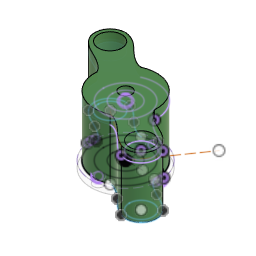
LED_clamp_fiber_mount_C20A10H740 v2 (Autodesk Fusion 360 design; units mm, degrees)
Autodesk Fusion 360 part; units mm, degrees
sketch "Sketch1" plane through (0, 0, 0) normal (0, 0, 1) x (1, 0, 0) in component "C20A1-H740-30"
  circle A0 centre (0, 0) radius 10
  line L0 (-10, 0) -> (10, 0) construction
  arc A1 (-9.9306, -1.1764) -> (-9.9306, 1.1764) centre (-10, 0) ccw
  line L1 (0, 0) -> (0, 5.1489) construction
  arc A2 (9.9306, 1.1764) -> (9.9306, -1.1764) centre (10, 0) ccw
  circle A3 centre (0, 7.8996) radius 1.5
  circle A4 centre (0, -7.8996) radius 1.5
  dimension "d4" = 20
  dimension "d8" = 3
  constraint coincident A0.centre L1.start
  constraint coincident A0 L0.start
  constraint coincident A0 L0.end
  constraint horizontal L0
  constraint coincident A0.centre L0
  constraint coincident A0 A1.start
  constraint coincident A0 A1.end
  constraint coincident L0.start A1.centre
  constraint perpendicular L0 L1
  constraint symmetric A1.start L1 A2.end
  constraint symmetric A1.end L1 A2.start
  constraint symmetric A1 L1 A2
  constraint coincident L1 A3.centre
  constraint symmetric L0 A3 A4
  measures "d4" diameter of A0
  measures "d8" diameter of A3
extrude "Extrude1" add sketch "Sketch1" along normal blind 1.9 contours A0 A1 A2 makes body 1 in component "C20A1-H740-30"
sketch "Sketch1 (2)" plane through (0, 0, 1.9) normal (0, 0, 1) x (-1, 0, 0) in component "optic fiber mount"
  circle A0 centre (0, -7.8996) radius 1.5 construction
  circle A1 centre (0, 7.8996) radius 1.5 construction
  arc A2 (9.9306, 1.1764) -> (-9.9306, 1.1764) centre (0, 0) ccw construction
  arc A3 (-9.9306, -1.1764) -> (-9.9306, 1.1764) centre (-10, 0) ccw construction
  arc A4 (-9.9306, -1.1764) -> (9.9306, -1.1764) centre (0, 0) ccw construction
  arc A5 (9.9306, 1.1764) -> (9.9306, -1.1764) centre (10, 0) ccw construction
  line L0 (12.7, -9.5942) -> (-12.7, -9.5942) construction
  line L1 (0, 0) -> (0, -1.0835) construction
  line L2 (0, -1.0835) -> (0, -4.3356) construction
  line L3 (0, 0) -> (-4.8971, 0) construction
  circle A6 centre (12.7, -9.5942) radius 3.429
  circle A7 centre (-12.7, -9.5942) radius 3.429
  circle A8 centre (0, 0) radius 1.8
  circle A9 centre (0, 0) radius 9
  circle A10 centre (0, 0) radius 6.46
  circle A11 centre (0, 0) radius 3.8
  spline S0 degree 5 poles (14.5589, -5.5565) (14.3535, -5.462) (13.9487, -5.267) (13.3592, -4.9569) (12.6123, -4.5075) (11.7634, -3.8821) (11.0225, -3.1882) (10.4081, -2.4217) (9.9244, -1.5822) (9.5489, -0.6771) (9.2444, 0.2825) (9.0258, 1.0848) (8.8613, 1.702) (8.7495, 2.12) (8.693, 2.3306) knots 0 0 0 0 0 0 0.1 0.2 0.3 0.4 0.5 0.6 0.7 0.8 0.9 1 1 1 1 1 1
  line L4 (0, 0) -> (12.7, -9.5942) construction
  spline S1 degree 5 poles (9.3242, -12.4858) (9.1771, -12.3141) (8.8789, -11.978) (8.4194, -11.4957) (7.783, -10.9001) (6.9494, -10.2544) (6.0795, -9.7314) (5.1742, -9.3499) (4.2345, -9.1141) (3.2612, -9.0002) (2.2549, -8.9696) (1.4234, -8.9786) (0.7847, -8.9891) (0.3521, -8.9958) (0.1341, -8.999) knots 0 0 0 0 0 0 0.1 0.2 0.3 0.4 0.5 0.6 0.7 0.8 0.9 1 1 1 1 1 1
  line L5 (15.6873, -6.0761) -> (13.4304, -5.037)
  line L6 (9.0147, 1.1306) -> (8.3713, 3.5305)
  line L7 (10.1323, -13.4293) -> (8.516, -11.5423)
  line L8 (1.3763, -8.9805) -> (-1.1081, -9.0175)
  arc A12 (9.3242, -12.4858) -> (14.5589, -5.5565) centre (12.7, -9.5942) ccw
  spline S2 degree 5 poles (-14.5589, -5.5565) (-14.3535, -5.462) (-13.9487, -5.267) (-13.3592, -4.9569) (-12.6123, -4.5075) (-11.7634, -3.8821) (-11.0225, -3.1882) (-10.4081, -2.4217) (-9.9244, -1.5822) (-9.5489, -0.6771) (-9.2444, 0.2825) (-9.0258, 1.0848) (-8.8613, 1.702) (-8.7495, 2.12) (-8.693, 2.3306) knots 0 0 0 0 0 0 0.1 0.2 0.3 0.4 0.5 0.6 0.7 0.8 0.9 1 1 1 1 1 1
  line L9 (-15.6873, -6.0761) -> (-13.4304, -5.037)
  line L10 (-9.0147, 1.1306) -> (-8.3713, 3.5305)
  spline S3 degree 5 poles (-9.3242, -12.4858) (-9.1771, -12.3141) (-8.8789, -11.978) (-8.4194, -11.4957) (-7.783, -10.9001) (-6.9494, -10.2544) (-6.0795, -9.7314) (-5.1742, -9.3499) (-4.2345, -9.1141) (-3.2612, -9.0002) (-2.2549, -8.9696) (-1.4234, -8.9786) (-0.7847, -8.9891) (-0.3521, -8.9958) (-0.1341, -8.999) knots 0 0 0 0 0 0 0.1 0.2 0.3 0.4 0.5 0.6 0.7 0.8 0.9 1 1 1 1 1 1
  line L11 (-10.1323, -13.4293) -> (-8.516, -11.5423)
  line L12 (-1.3763, -8.9805) -> (1.1081, -9.0175)
  arc A13 (-14.5589, -5.5565) -> (-9.3242, -12.4858) centre (-12.7, -9.5942) ccw
  point P0 (0, -9.5942)
  point P1 (10.4158, -2.3671)
  point P2 (5.1238, -9.3722)
  point P3 (-10.4158, -2.3671)
  point P4 (-5.1238, -9.3722)
  dimension "d17" = 25.4
  dimension "d18" = 6.858
  dimension "d19" = 6.858
  dimension "d24" = 3.6
  dimension "d26" = 18
  dimension "d30" = 2
  dimension "d31" = 8.89
  constraint coincident A2.centre A4.centre
  constraint horizontal L0
  constraint midpoint L0 P0
  constraint vertical L1
  constraint parallel L1 L2
  constraint perpendicular L1 L3
  constraint coincident P0 L2
  constraint coincident L0.start A6.centre
  constraint coincident L0.end A7.centre
  constraint concentric A8 A9
  constraint concentric A6 A12
  constraint coincident A9 S0.end
  constraint tangent A9 S0
  constraint tangent S0 A12
  constraint midpoint S0.start L5
  constraint midpoint S0.end L6
  constraint symmetric S0.start L4 S1.start
  constraint symmetric P1 L4 P2
  constraint symmetric S0.end L4 S1.end
  constraint symmetric L4 L5.start L7.start
  constraint symmetric L4 L5.end L7.end
  constraint symmetric L4 L6.start L8.start
  constraint symmetric L4 L6.end L8.end
  constraint symmetric L2 S0.start S2.start
  constraint symmetric L2 P1 P3
  constraint symmetric L2 S0.end S2.end
  constraint symmetric L2 S1.start S3.start
  constraint symmetric L2 P2 P4
  constraint symmetric L2 S1.end S3.end
  constraint symmetric L2 L5.start L9.start
  constraint symmetric L2 L5.end L9.end
  constraint symmetric L2 L6.start L10.start
  constraint symmetric L2 L6.end L10.end
  constraint symmetric L2 L7.start L11.start
  constraint symmetric L2 L7.end L11.end
  constraint symmetric L2 L8.start L12.start
  constraint symmetric L2 L8.end L12.end
  constraint symmetric L2 A12 A13
  measures "d17" distance of L0.start L0.end
  measures "d18" diameter of A6
  measures "d19" diameter of A7
  measures "d24" diameter of A8
  measures "d26" diameter of A9
  measures "d31" diameter of A12
extrude "Extrude1'" add sketch "Sketch1 (2)" along normal blind 15 separate body contours A9 L8 L12 | A9 S0 S1 L6 L8 A12 | A9 S2 L10 S3 L12 A13 makes body 2 in component "optic fiber mount"
sketch "Sketch2" plane through (0, 0, 0) normal (1, 0, 0) x (0, 1, 0) in component "optic fiber mount"
  line L0 (1.1764, 1.9) -> (-1.1764, 1.9)
  line L1 (1.1764, 1.9) -> (-1.1764, 1.9)
  line L2 (-1.1764, 1.9) -> (1.1764, 1.9) construction
  arc A0 (2.5, 1.9) -> (-2.5, 1.9) centre (0, 1.9) ccw
  line L3 (-2.5, 1.9) -> (2.5, 1.9)
  point P0 (0, 1.9)
  dimension "d36" = 5
  constraint coincident L0.end L1.end
  constraint coincident L0.start L1.start
  constraint midpoint L2 P0
  constraint coincident P0 A0.centre
  constraint parallel L2 L3
  constraint coincident L0.end L3
  measures "d36" distance of A0.start A0.end
extrude "Extrude2" cut sketch "Sketch2" along normal mid plane 43.18 bodies 2 in component "optic fiber mount"
sketch "Sketch3" plane through (0, 0, 16.9) normal (0, 0, 1) x (-1, 0, 0) in component "optic fiber mount"
  circle A0 centre (0, 0) radius 6.46
  circle A1 centre (-12.7, -9.5942) radius 3.429
  circle A2 centre (12.7, -9.5942) radius 3.429
  arc A3 (9.3242, -12.4858) -> (14.5589, -5.5565) centre (12.7, -9.5942) ccw
  spline S0 degree 5 poles (14.5589, -5.5565) (14.3535, -5.462) (13.9487, -5.267) (13.3592, -4.9569) (12.6123, -4.5075) (11.7634, -3.8821) (11.0225, -3.1882) (10.4081, -2.4217) (9.9244, -1.5822) (9.5489, -0.6771) (9.2444, 0.2825) (9.0258, 1.0848) (8.8613, 1.702) (8.7495, 2.12) (8.693, 2.3306) knots 0 0 0 0 0 0 0.1 0.2 0.3 0.4 0.5 0.6 0.7 0.8 0.9 1 1 1 1 1 1
  arc A4 (8.693, 2.3306) -> (-8.693, 2.3306) centre (0, 0) ccw
  spline S1 degree 5 poles (-8.693, 2.3306) (-8.7495, 2.12) (-8.8613, 1.702) (-9.0258, 1.0848) (-9.2444, 0.2825) (-9.5489, -0.6771) (-9.9244, -1.5822) (-10.4081, -2.4217) (-11.0225, -3.1882) (-11.7634, -3.8821) (-12.6123, -4.5075) (-13.3592, -4.9569) (-13.9487, -5.267) (-14.3535, -5.462) (-14.5589, -5.5565) knots -1 -1 -1 -1 -1 -1 -0.9 -0.8 -0.7 -0.6 -0.5 -0.4 -0.3 -0.2 -0.1 0 0 0 0 0 0
  arc A5 (-14.5589, -5.5565) -> (-9.3242, -12.4858) centre (-12.7, -9.5942) ccw
  spline S2 degree 5 poles (-9.3242, -12.4858) (-9.1771, -12.3141) (-8.8789, -11.978) (-8.4194, -11.4957) (-7.783, -10.9001) (-6.9494, -10.2544) (-6.0795, -9.7314) (-5.1742, -9.3499) (-4.2345, -9.1141) (-3.2612, -9.0002) (-2.2549, -8.9696) (-1.4234, -8.9786) (-0.7847, -8.9891) (-0.3521, -8.9958) (-0.1341, -8.999) knots 0 0 0 0 0 0 0.1 0.2 0.3 0.4 0.5 0.6 0.7 0.8 0.9 1 1 1 1 1 1
  arc A6 (-0.1341, -8.999) -> (0.1341, -8.999) centre (0, 0) ccw
  spline S3 degree 5 poles (0.1341, -8.999) (0.3521, -8.9958) (0.7847, -8.9891) (1.4234, -8.9786) (2.2549, -8.9696) (3.2612, -9.0002) (4.2345, -9.1141) (5.1742, -9.3499) (6.0795, -9.7314) (6.9494, -10.2544) (7.783, -10.9001) (8.4194, -11.4957) (8.8789, -11.978) (9.1771, -12.3141) (9.3242, -12.4858) knots -1 -1 -1 -1 -1 -1 -0.9 -0.8 -0.7 -0.6 -0.5 -0.4 -0.3 -0.2 -0.1 0 0 0 0 0 0
  circle A7 centre (0, 0) radius 3.8
  circle A8 centre (0, 0) radius 1.8
extrude "Extrude3" add sketch "Sketch3" along normal blind 2.54 contours A0 | A3 S0 A4 S1 A5 S2 A6 S3 | A7 bodies 2 in component "optic fiber mount"
extrude "Extrude4" add sketch "Sketch3" against normal blind 10 contours A7 bodies 2 in component "optic fiber mount"
sketch "Sketch1 (3)" plane through (0, 0, 1.9) normal (0, 0, 1) x (-1, 0, 0) in component "optic fiber mount_v2"
  circle A0 centre (0, -7.8996) radius 1.5 construction
  circle A1 centre (0, 7.8996) radius 1.5 construction
  arc A2 (9.9306, 1.1764) -> (-9.9306, 1.1764) centre (0, 0) ccw construction
  arc A3 (-9.9306, -1.1764) -> (-9.9306, 1.1764) centre (-10, 0) ccw construction
  arc A4 (-9.9306, -1.1764) -> (9.9306, -1.1764) centre (0, 0) ccw construction
  arc A5 (9.9306, 1.1764) -> (9.9306, -1.1764) centre (10, 0) ccw construction
  line L0 (0, 0) -> (0, -1.0835) construction
  line L1 (0, -1.0835) -> (0, -4.3356) construction
  line L2 (0, 0) -> (-4.8971, 0) construction
  circle A6 centre (14.7588, -10.2352) radius 3.429
  circle A7 centre (0, 0) radius 1.8
  circle A8 centre (0, 0) radius 9
  circle A9 centre (0, 0) radius 6.46
  circle A10 centre (0, 0) radius 3.8
  spline S0 degree 5 poles (18.0452, -7.2423) (17.8661, -7.0456) (17.5068, -6.6748) (16.9644, -6.1863) (16.231, -5.6579) (15.2794, -5.1336) (14.2775, -4.6622) (13.2223, -4.1647) (12.1352, -3.5856) (11.0769, -2.9147) (10.1307, -2.171) (9.5326, -1.5431) (9.2055, -1.0673) (9.0458, -0.7499) (8.9806, -0.5911) knots 0 0 0 0 0 0 0.1 0.2 0.3 0.4 0.5 0.6 0.7 0.8 0.9 1 1 1 1 1 1
  line L3 (0, 0) -> (14.7588, -10.2352) construction
  spline S1 degree 5 poles (13.1077, -14.3622) (12.8607, -14.2633) (12.3874, -14.0567) (11.7398, -13.72) (10.9878, -13.2183) (10.1633, -12.5109) (9.3706, -11.7377) (8.5348, -10.9238) (7.6114, -10.1087) (6.6122, -9.3527) (5.584, -8.7271) (4.7863, -8.3871) (4.226, -8.2475) (3.8728, -8.2092) (3.7012, -8.2037) knots 0 0 0 0 0 0 0.1 0.2 0.3 0.4 0.5 0.6 0.7 0.8 0.9 1 1 1 1 1 1
  line L4 (18.9294, -8.2133) -> (17.1611, -6.2714)
  line L5 (9.303, -1.3755) -> (8.6581, 0.1933)
  line L6 (14.3269, -14.8499) -> (11.8884, -13.8744)
  line L7 (4.5489, -8.2308) -> (2.8536, -8.1767)
  arc A11 (13.1077, -14.3622) -> (18.0452, -7.2423) centre (14.7588, -10.2352) ccw
  line L8 (0, 0) -> (-11.1406, -16.0644) construction
  spline S2 degree 5 poles (-18.0452, 7.2423) (-17.8661, 7.0456) (-17.5068, 6.6748) (-16.9644, 6.1863) (-16.231, 5.6579) (-15.2794, 5.1336) (-14.2775, 4.6622) (-13.2223, 4.1647) (-12.1352, 3.5856) (-11.0769, 2.9147) (-10.1307, 2.171) (-9.5326, 1.5431) (-9.2055, 1.0673) (-9.0458, 0.7499) (-8.9806, 0.5911) knots 0 0 0 0 0 0 0.1 0.2 0.3 0.4 0.5 0.6 0.7 0.8 0.9 1 1 1 1 1 1
  line L9 (-18.9294, 8.2133) -> (-17.1611, 6.2714)
  line L10 (-9.303, 1.3755) -> (-8.6581, -0.1933)
  arc A12 (-13.1077, 14.3622) -> (-18.0452, 7.2423) centre (-14.7588, 10.2352) ccw
  circle A13 centre (-14.7588, 10.2352) radius 3.429
  spline S3 degree 5 poles (-13.1077, 14.3622) (-12.8607, 14.2633) (-12.3874, 14.0567) (-11.7398, 13.72) (-10.9878, 13.2183) (-10.1633, 12.5109) (-9.3706, 11.7377) (-8.5348, 10.9238) (-7.6114, 10.1087) (-6.6122, 9.3527) (-5.584, 8.7271) (-4.7863, 8.3871) (-4.226, 8.2475) (-3.8728, 8.2092) (-3.7012, 8.2037) knots 0 0 0 0 0 0 0.1 0.2 0.3 0.4 0.5 0.6 0.7 0.8 0.9 1 1 1 1 1 1
  line L11 (-14.3269, 14.8499) -> (-11.8884, 13.8744)
  line L12 (-4.5489, 8.2308) -> (-2.8536, 8.1767)
  point P0 (0, -9.5942)
  point P1 (13.1402, -4.1068)
  point P2 (8.4518, -10.8672)
  point P3 (-13.1402, 4.1068)
  point P4 (-8.4518, 10.8672)
  dimension "d18_1" = 6.858
  dimension "d24_1" = 3.6
  dimension "d26_1" = 18
  dimension "d30_1" = 2
  dimension "d31_1" = 8.89
  dimension "d43" = 17.9605
  constraint coincident A2.centre A4.centre
  constraint vertical L0
  constraint parallel L0 L1
  constraint perpendicular L0 L2
  constraint coincident P0 L1
  constraint concentric A7 A8
  constraint concentric A6 A11
  constraint coincident A8 S0.end
  constraint tangent S0 A11
  constraint coincident A6.centre L3.end
  constraint midpoint S0.start L4
  constraint midpoint S0.end L5
  constraint symmetric S0.start L3 S1.start
  constraint symmetric P1 L3 P2
  constraint symmetric S0.end L3 S1.end
  constraint symmetric L3 L4.start L6.start
  constraint symmetric L3 L4.end L6.end
  constraint symmetric L3 L5.start L7.start
  constraint symmetric L3 L5.end L7.end
  constraint perpendicular L3 L8
  constraint coincident A5 S0.end
  constraint symmetric A6 L8 A13
  constraint symmetric S0.start L8 A12.start
  constraint symmetric P1 L8 P4
  constraint symmetric S0.end L8 S3.end
  constraint symmetric S1.start L8 S2.start
  constraint symmetric P2 L8 P3
  constraint symmetric S1.end L8 S2.end
  constraint symmetric L4.start L8 L11.start
  constraint symmetric L4.end L8 L11.end
  constraint symmetric L5.start L8 L12.start
  constraint symmetric L5.end L8 L12.end
  constraint symmetric L6.start L8 L9.start
  constraint symmetric L6.end L8 L9.end
  constraint symmetric L7.start L8 L10.start
  constraint symmetric L7.end L8 L10.end
  constraint symmetric A11 L8 A12
  measures "d18_1" diameter of A6
  measures "d24_1" diameter of A7
  measures "d26_1" diameter of A8
  measures "d31_1" diameter of A11
  measures "d43" distance of A2.centre A6.centre
extrude "Extrude1''" add sketch "Sketch1 (3)" along normal blind 15 separate body contours A8 | A8 S2 A12 S3 | A8 S0 S1 A11 makes body 3 in component "optic fiber mount_v2"
sketch "Sketch2 (2)" plane through (0, 0, 0) normal (1, 0, 0) x (0, 1, 0) in component "optic fiber mount_v2"
  line L0 (1.1764, 1.9) -> (-1.1764, 1.9)
  line L1 (1.1764, 1.9) -> (-1.1764, 1.9)
  line L2 (-1.1764, 1.9) -> (1.1764, 1.9) construction
  arc A0 (2.5, 1.9) -> (-2.5, 1.9) centre (0, 1.9) ccw
  line L3 (-2.5, 1.9) -> (2.5, 1.9)
  point P0 (0, 1.9)
  dimension "d36_1" = 5
  constraint coincident L0.end L1.end
  constraint coincident L0.start L1.start
  constraint midpoint L2 P0
  constraint coincident P0 A0.centre
  constraint parallel L2 L3
  constraint coincident L0.end L3
  measures "d36_1" distance of A0.start A0.end
extrude "Extrude2'" cut sketch "Sketch2 (2)" along normal mid plane 43.18 bodies 3 in component "optic fiber mount_v2"
sketch "Sketch3 (2)" plane through (0, 0, 16.9) normal (0, 0, 1) x (-1, 0, 0) in component "optic fiber mount_v2"
  circle A0 centre (14.7588, -10.2352) radius 3.429
  arc A1 (13.1077, -14.3622) -> (18.0452, -7.2423) centre (14.7588, -10.2352) ccw
  spline S0 degree 5 poles (18.0452, -7.2423) (17.8661, -7.0456) (17.5068, -6.6748) (16.9644, -6.1863) (16.231, -5.6579) (15.2794, -5.1336) (14.2775, -4.6622) (13.2223, -4.1647) (12.1352, -3.5856) (11.0769, -2.9147) (10.1307, -2.171) (9.5326, -1.5431) (9.2055, -1.0673) (9.0458, -0.7499) (8.9806, -0.5911) knots 0 0 0 0 0 0 0.1 0.2 0.3 0.4 0.5 0.6 0.7 0.8 0.9 1 1 1 1 1 1
  arc A2 (8.9806, -0.5911) -> (-3.7012, 8.2037) centre (0, 0) ccw
  spline S1 degree 5 poles (3.7012, -8.2037) (3.8728, -8.2092) (4.226, -8.2475) (4.7863, -8.3871) (5.584, -8.7271) (6.6122, -9.3527) (7.6114, -10.1087) (8.5348, -10.9238) (9.3706, -11.7377) (10.1633, -12.5109) (10.9878, -13.2183) (11.7398, -13.72) (12.3874, -14.0567) (12.8607, -14.2633) (13.1077, -14.3622) knots -1 -1 -1 -1 -1 -1 -0.9 -0.8 -0.7 -0.6 -0.5 -0.4 -0.3 -0.2 -0.1 0 0 0 0 0 0
  circle A3 centre (0, 0) radius 3.8
  circle A4 centre (0, 0) radius 1.8
  circle A5 centre (-14.7588, 10.2352) radius 3.429
  circle A6 centre (0, 0) radius 6.46
  spline S2 degree 5 poles (-18.0452, 7.2423) (-17.8661, 7.0456) (-17.5068, 6.6748) (-16.9644, 6.1863) (-16.231, 5.6579) (-15.2794, 5.1336) (-14.2775, 4.6622) (-13.2223, 4.1647) (-12.1352, 3.5856) (-11.0769, 2.9147) (-10.1307, 2.171) (-9.5326, 1.5431) (-9.2055, 1.0673) (-9.0458, 0.7499) (-8.9806, 0.5911) knots 0 0 0 0 0 0 0.1 0.2 0.3 0.4 0.5 0.6 0.7 0.8 0.9 1 1 1 1 1 1
  arc A7 (-8.9806, 0.5911) -> (3.7012, -8.2037) centre (0, 0) ccw
  spline S3 degree 5 poles (-3.7012, 8.2037) (-3.8728, 8.2092) (-4.226, 8.2475) (-4.7863, 8.3871) (-5.584, 8.7271) (-6.6122, 9.3527) (-7.6114, 10.1087) (-8.5348, 10.9238) (-9.3706, 11.7377) (-10.1633, 12.5109) (-10.9878, 13.2183) (-11.7398, 13.72) (-12.3874, 14.0567) (-12.8607, 14.2633) (-13.1077, 14.3622) knots -1 -1 -1 -1 -1 -1 -0.9 -0.8 -0.7 -0.6 -0.5 -0.4 -0.3 -0.2 -0.1 0 0 0 0 0 0
  arc A8 (-13.1077, 14.3622) -> (-18.0452, 7.2423) centre (-14.7588, 10.2352) ccw
extrude "Extrude3'" add sketch "Sketch3 (2)" along normal blind 2.54 contours A1 S0 A2 S1 S2 A7 S3 A8 | A3 | A6 bodies 3 in component "optic fiber mount_v2"
extrude "Extrude4'" add sketch "Sketch3 (2)" against normal blind 10 contours A3 bodies 3 in component "optic fiber mount_v2"
component "C20A1-H740-30" placed x (1, 0, 0) y (0, 1, 0) z (0, 0, 1) at (0, 0, 0)
component "optic fiber mount" placed x (1, 0, 0) y (0, 1, 0) z (0, 0, 1) at (0, 0, 0)
component "optic fiber mount_v2" placed x (1, 0, 0) y (0, 1, 0) z (0, 0, 1) at (0, 0, 0)
equation "C20A1_H740_30_diam = 20 mm"
equation "C20A1_H740_30_thick = 1.9 mm"
equation "C20A1_H740_30_holes_dist = 15 mm"
equation "d4 = C20A1_H740_30_diam"
equation "d5 = C20A1_H740_30_thick"
equation "C20A1_H740_30_holes_diam = 3 mm"
equation "d8 = C20A1_H740_30_holes_diam"
equation "screw_1_4_20_free_fit = 0.27 in"
equation "screw_1_4_20_free_tap = 0.201 in"
equation "screw_1_4_20_cap_diam = 0.3 in"
equation "mount_clamp_screw_free_fit = screw_1_4_20_free_fit"
equation "mount_clamp_screw_cap_diam = screw_1_4_20_cap_diam"
equation "mount_clamp_screw_dist = 1 in"
equation "mount_clamp_screw_diam = 0.25 in"
equation "d17 = mount_clamp_screw_dist"
equation "d18 = mount_clamp_screw_free_fit"
equation "d19 = mount_clamp_screw_free_fit"
equation "mount_clamp_thick = 0.12 in"
equation "optic_fiber_diam = 3 mm"
equation "mount_clamp_walls_thick = 0.1 in"
equation "optic_fiber_elevation = 5 mm"
equation "d24 = optic_fiber_hole_diam"
equation "mount_clamp_diam = C20A1_H740_30_diam - 2 mm"
equation "d26 = mount_clamp_diam"
equation "d27 = -mount_clamp_walls_thick"
equation "mount_clamp_height = 15 mm"
equation "optic_fiber_wall_thick = 2 mm"
equation "d30 = optic_fiber_wall_thick"
equation "d32 = mount_clamp_height"
equation "d37 = mount_clamp_walls_thick"
equation "d39 = -mount_clamp_height + optic_fiber_elevation"
equation "optic_fiber_plastic_clearance = 0.3 mm"
equation "optic_fiber_hole_diam = optic_fiber_diam + optic_fiber_plastic_clearance * 2"
equation "d18_1 = mount_clamp_screw_free_fit"
equation "d24_1 = optic_fiber_hole_diam"
equation "d26_1 = mount_clamp_diam"
equation "d27_1 = -mount_clamp_walls_thick"
equation "d30_1 = optic_fiber_wall_thick"
equation "d32_1 = mount_clamp_height"
equation "d37_1 = mount_clamp_walls_thick"
equation "d39_1 = -mount_clamp_height + optic_fiber_elevation"
equation "d43 = ( sqrt(2) / 2 ) * 1 in"
named bodies: "LED_clamp_fiber_mount_C20A10H740_3mm_v1"
